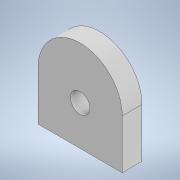
# Autodesk Inventor part: Soporte
Saved by Autodesk Inventor 2022 (Build 260153000, 153)
## iProperties
Created: 2022-01-11
Part Number: Soporte
Material: Generic
Document SubType Name: Modeling
Designer: Yeison
Density: 1 g/cm^3
Appearance: Default
Author: Yeison
Autodesk Inventor part; units mm, degrees
ref_plane "YZ Plane" through (0, 0, 0) normal (1, 0, 0) x (0, 1, 0)
ref_plane "XZ Plane" through (0, 0, 0) normal (0, 1, 0) x (-1, 0, 0)
ref_plane "XY Plane" through (0, 0, 0) normal (0, 0, 1) x (1, 0, 0)
sketch "Sketch1" plane through (0, 0, 0) normal (0, 0, 1) x (1, 0, 0)
  circle A0 centre (0, 0) radius 5.5
  line L0 (5.5, 0) -> (23.5, 0)
  line L1 (-5.5, 0) -> (-23.5, 0)
  line L2 (-23.5, 0) -> (-23.5, 5.5)
  line L3 (23.5, 0) -> (23.5, 5.5)
  arc A1 (23.5, 5.5) -> (-23.5, 5.5) centre (0, 5.5) ccw
  line L4 (-23.5, 0) -> (-23.5, -22)
  line L5 (-23.5, -22) -> (23.5, -22)
  line L6 (23.5, -22) -> (23.5, 0)
  dimension "d0" = 11
  dimension "d1" = 18
  dimension "d2" = 18
  dimension "d3" = 22
  constraints: 14 end point, 5 point on circle, 3 vertical, 2 centre point, 2 horizontal, 2 perpendicular, 1 coincident
  measures "d0" diameter of A0
  measures "d1" distance of L0.start L0.end
  measures "d2" distance of L1.start L1.end
  measures "d3" distance of L1.end L4.end
extrude "Extrusion1" add sketch "Sketch1" along normal blind 10 and the other way blind 1 contours L0 L6 L5 L4 L1 A0 | A0 L1 L2 A1 L3 L0
sketch "Sketch2" plane through (0, 0, -1) normal (0, 0, -1) x (-1, 0, 0)
  circle A0 centre (0, 0) radius 5.5
  constraints: 1 centre point, 1 coincident
extrude "Extrusion2" add sketch "Sketch2" against normal blind 1
body "Solid1"
